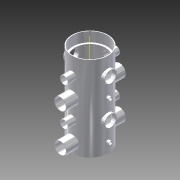
# Autodesk Inventor part: Detection Region Vacuum Collar v2
Saved by Autodesk Inventor 2015 SP1 (Build 190203100, 203)
## iProperties
Created: 2014-06-20
Part Number: Detection Region Vacuum Collar v2
Material: Aluminum 6061-AHC
Document SubType Name: Modeling
Designer: Aki
Density: 2.7 g/cm^3
Appearance: Aluminum - Dark
Author: Aki
Autodesk Inventor part; units mm, degrees
sketch "Sketch1" plane through (0, 0, 0) normal (0, 1, 0) x (-1, 0, 0)
  circle A0 centre (0, 0) radius 101.6
  circle A1 centre (0, 0) radius 97.6
  dimension "d0" = 203.2
  dimension "d3" = 195.2
  constraints: 2 centre point, 2 coincident
  measures "d0" diameter of A0
  measures "d3" diameter of A1
extrude "Extrusion2" add sketch "Sketch1" along normal blind 477.1
ref_plane "Work Plane1" through (0, 0, 101.6) normal (0, 0, 1) x (1, 0, 0)
sketch "Sketch2" plane through (0, 0, 101.6) normal (0, 0, 1) x (1, 0, 0)
  circle A0 centre (0, 57.3) radius 35.05
  circle A1 centre (0, 164.8) radius 22.25
  circle A2 centre (0, 272.3) radius 35.05
  circle A3 centre (0, 379.8) radius 22.25
  line L0 (101.6, 477.1) -> (-101.6, 477.1) projected
  line L1 (-101.6, 0) -> (101.6, 0) projected
  point P0 (0, 0)
  dimension "d7" = 70.1
  dimension "d8" = 44.5
  dimension "d9" = 70.1
  dimension "d10" = 44.5
  dimension "d11" = 97.3
  dimension "d12" = 57.3
  dimension "d13" = 215
  dimension "d14" = 215
  constraints: 4 centre point
  measures "d7" diameter of A0
  measures "d8" diameter of A1
  measures "d9" diameter of A2
  measures "d10" diameter of A3
  measures "d11" distance from line of L0 A3.centre
  measures "d12" distance from line of L1 A0.centre
  measures "d13" distance of A2.centre A0.centre
  measures "d14" distance of A3.centre A1.centre
extrude "Extrusion8" add sketch "Sketch2" against normal up to next
sketch "Sketch13" plane through (0, 0, 101.6) normal (0, 0, 1) x (1, 0, 0)
  circle A0 centre (0, 57.3) radius 35.05
  circle A1 centre (0, 164.8) radius 22.25
  circle A2 centre (0, 272.3) radius 35.05
  circle A3 centre (0, 379.8) radius 22.25
  line L0 (101.6, 477.1) -> (-101.6, 477.1) projected
  line L1 (-101.6, 0) -> (101.6, 0) projected
  point P0 (0, 0)
  dimension "d104" = 70.1
  dimension "d105" = 44.5
  dimension "d106" = 70.1
  dimension "d107" = 44.5
  dimension "d108" = 97.3
  dimension "d109" = 57.3
  dimension "d110" = 215
  dimension "d111" = 215
  constraints: 4 centre point
  measures "d104" diameter of A0
  measures "d105" diameter of A1
  measures "d106" diameter of A2
  measures "d107" diameter of A3
  measures "d108" distance from line of L0 A3.centre
  measures "d109" distance from line of L1 A0.centre
  measures "d110" distance of A2.centre A0.centre
  measures "d111" distance of A3.centre A1.centre
extrude "Extrusion9" add sketch "Sketch13" along normal blind 65
ref_plane "Work Plane2" through (0, 0, -101.6) normal (0, 0, 1) x (1, 0, 0)
sketch "Sketch3" plane through (0, 0, -101.6) normal (0, 0, 1) x (1, 0, 0)
  circle A0 centre (0, 57.3) radius 35.05
  circle A1 centre (0, 164.8) radius 22.25
  circle A2 centre (0, 272.3) radius 35.05
  circle A3 centre (0, 379.8) radius 22.25
  line L0 (101.6, 477.1) -> (-101.6, 477.1) projected
  line L1 (-101.6, 0) -> (101.6, 0) projected
  line L2 (0, 357.55) -> (0, 402.05) projected
  point P0 (0, 0)
  dimension "d18" = 70.1
  dimension "d19" = 44.5
  dimension "d20" = 70.1
  dimension "d21" = 44.5
  dimension "d22" = 97.3
  dimension "d23" = 57.3
  dimension "d24" = 215
  dimension "d25" = 215
  dimension "d26" = 0
  constraints: 4 centre point
  measures "d18" diameter of A0
  measures "d19" diameter of A1
  measures "d20" diameter of A2
  measures "d21" diameter of A3
  measures "d22" distance from line of L0 A3.centre
  measures "d23" distance from line of L1 A0.centre
  measures "d24" distance of A0.centre A2.centre
  measures "d25" distance of A3.centre A1.centre
  measures "d26" distance from line of L2 A3.centre
extrude "Extrusion10" add sketch "Sketch3" along normal up to next
sketch "Sketch14" plane through (0, 0, -101.6) normal (0, 0, 1) x (1, 0, 0)
  circle A0 centre (0, 57.3) radius 35.05
  circle A1 centre (0, 164.8) radius 22.25 projected
  circle A2 centre (0, 164.8) radius 22.25
  circle A3 centre (0, 272.3) radius 35.05
  circle A4 centre (0, 379.8) radius 22.25
  line L0 (-101.6, 0) -> (101.6, 0) projected
  line L1 (101.6, 477.1) -> (-101.6, 477.1) projected
  point P0 (0, 0)
  dimension "d116" = 70.1
  dimension "d117" = 44.5
  dimension "d118" = 70.1
  dimension "d119" = 44.5
  dimension "d120" = 57.3
  dimension "d121" = 215
  dimension "d122" = 215
  dimension "d123" = 97.3
  constraints: 4 centre point, 1 coincident
  measures "d116" diameter of A0
  measures "d117" diameter of A2
  measures "d118" diameter of A3
  measures "d119" diameter of A4
  measures "d120" distance from line of L0 A0.centre
  measures "d121" distance of A3.centre A0.centre
  measures "d122" distance of A4.centre A2.centre
  measures "d123" distance from line of L1 A4.centre
extrude "Extrusion11" add sketch "Sketch14" against normal blind 65
sketch "Sketch15" plane through (0, 379.8, -166.6) normal (0, 0, -1) x (-1, 0, 0)
  circle A0 centre (0, -322.5106) radius 34.15
  point P0 (0, -379.8)
  dimension "d126" = 68.3
  constraints: 1 centre point
  measures "d126" diameter of A0
hole "Hole8" at (0, 57.2894, -166.6) direction (0, 0, 1) diameter 61.976 end through all
sketch "Sketch16" plane through (0, 164.8, -166.6) normal (0, 0, -1) x (-1, 0, 0)
  circle A0 centre (0, 0) radius 21.35
  point P0 (0, -164.8)
  dimension "d134" = 42.7
  constraints: 1 centre point
  measures "d134" diameter of A0
hole "Hole9" at (0, 164.8, -166.6) direction (0, 0, 1) diameter 42.7 end through all
sketch "Sketch17" plane through (0, 272.3, -166.6) normal (0, 0, -1) x (-1, 0, 0)
  circle A0 centre (0, 0) radius 34.15
  point P0 (0, -272.3)
  dimension "d142" = 68.3
  constraints: 1 centre point
  measures "d142" diameter of A0
hole "Hole10" at (0, 272.3, -166.6) direction (0, 0, 1) diameter 61.976 end through all
sketch "Sketch18" plane through (0, 379.8, -166.6) normal (0, 0, -1) x (-1, 0, 0)
  circle A0 centre (0, 0) radius 21.35
  point P0 (0, -379.8)
  dimension "d150" = 42.7
  constraints: 1 centre point
  measures "d150" diameter of A0
hole "Hole11" at (0, 379.8, -166.6) direction (0, 0, 1) diameter 42.7 end through all
ref_plane "Work Plane3" through (101.6, 0, 0) normal (1, 0, 0) x (0, 1, 0)
sketch "Sketch27" plane through (101.6, 0, 0) normal (1, 0, 0) x (0, 1, 0)
  circle A0 centre (164.8, 0) radius 35.05
  circle A1 centre (379.8, 0) radius 35.05
  line L0 (477.1, -101.6) -> (477.1, 101.6) projected
  circle A2 centre (272.3, 0) radius 9.65
  circle A3 centre (57.3, 0) radius 9.65
  point P0 (0, 0)
  dimension "d204" = 70.1
  dimension "d205" = 70.1
  dimension "d206" = 97.3
  dimension "d207" = 215
  dimension "d208" = 19.3
  dimension "d209" = 19.3
  dimension "d210" = 215
  dimension "d211" = 107.5
  constraints: 4 centre point
  measures "d204" diameter of A0
  measures "d205" diameter of A1
  measures "d206" distance from line of L0 A1.centre
  measures "d207" distance of A0.centre A1.centre
  measures "d208" diameter of A2
  measures "d209" diameter of A3
  measures "d210" distance of A3.centre A2.centre
  measures "d211" distance of A2.centre A1.centre
extrude "Extrusion17" add sketch "Sketch27" against normal up to next
sketch "Sketch28" plane through (101.6, 0, 0) normal (1, 0, 0) x (0, 1, 0)
  circle A0 centre (57.3, 0) radius 9.65
  circle A1 centre (272.3, 0) radius 9.65
  circle A2 centre (164.8, 0) radius 35.05
  circle A3 centre (379.8, 0) radius 35.05
  line L0 (477.1, -101.6) -> (477.1, 101.6) projected
  point P0 (0, 0)
  dimension "d214" = 19.3
  dimension "d215" = 19.3
  dimension "d216" = 70.1
  dimension "d217" = 70.1
  dimension "d218" = 97.3
  dimension "d219" = 107.5
  dimension "d220" = 215
  dimension "d221" = 215
  constraints: 4 centre point
  measures "d214" diameter of A0
  measures "d215" diameter of A1
  measures "d216" diameter of A2
  measures "d217" diameter of A3
  measures "d218" distance from line of L0 A3.centre
  measures "d219" distance of A1.centre A3.centre
  measures "d220" distance of A2.centre A3.centre
  measures "d221" distance of A1.centre A0.centre
extrude "Extrusion18" add sketch "Sketch28" along normal blind 15
ref_plane "Work Plane8" through (-101.6, 0, 0) normal (1, 0, 0) x (0, 1, 0)
sketch "Sketch33" plane through (-101.6, 0, 0) normal (1, 0, 0) x (0, 1, 0)
  circle A0 centre (164.8, 0) radius 35.05
  circle A1 centre (379.8, 0) radius 35.05
  line L0 (477.1, -101.6) -> (477.1, 101.6) projected
  circle A2 centre (272.3, 0) radius 9.515
  circle A3 centre (57.3, 0) radius 9.65 projected
  circle A4 centre (57.3, 0) radius 9.65
  point P0 (0, 0)
  dimension "d230" = 70.1
  dimension "d231" = 70.1
  dimension "d232" = 97.3
  dimension "d233" = 215
  dimension "d234" = 19.03
  dimension "d235" = 107.5
  dimension "d236" = 19.3
  dimension "d237" = 215
  constraints: 4 centre point, 1 coincident
  measures "d230" diameter of A0
  measures "d231" diameter of A1
  measures "d232" distance from line of L0 A1.centre
  measures "d233" distance of A0.centre A1.centre
  measures "d234" diameter of A2
  measures "d235" distance of A1.centre A2.centre
  measures "d236" diameter of A4
  measures "d237" distance of A2.centre A4.centre
extrude "Extrusion19" add sketch "Sketch33" along normal up to next
sketch "Sketch34" plane through (-101.6, 0, 0) normal (1, 0, 0) x (0, 1, 0)
  circle A0 centre (379.8, 0) radius 35.05
  circle A1 centre (164.8, 0) radius 35.05
  line L0 (477.1, -101.6) -> (477.1, 101.6) projected
  arc A2 (262.785, 0) -> (281.815, 0) centre (272.3, 0) ccw projected
  circle A3 centre (272.3, 0) radius 9.65
  arc A4 (47.65, 0) -> (66.95, 0) centre (57.3, 0) ccw projected
  circle A5 centre (57.3, 0) radius 9.65
  point P0 (0, 0)
  point P1 (312.785, 0)
  point P2 (331.815, 0)
  point P3 (97.65, 0)
  point P4 (116.95, 0)
  point P5 (252.785, 0)
  point P6 (271.815, 0)
  point P7 (37.65, 0)
  point P8 (56.95, 0)
  dimension "d240" = 70.1
  dimension "d241" = 70.1
  dimension "d242" = 97.3
  dimension "d243" = 215
  dimension "d244" = 19.3
  dimension "d245" = 19.3
  dimension "d246" = 107.5
  dimension "d247" = 215
  constraints: 4 centre point, 2 coincident, 2 other
  measures "d240" diameter of A0
  measures "d241" diameter of A1
  measures "d242" distance from line of L0 A0.centre
  measures "d243" distance of A1.centre A0.centre
  measures "d244" diameter of A3
  measures "d245" diameter of A5
  measures "d246" distance of A3.centre A0.centre
  measures "d247" distance of A5.centre A3.centre
extrude "Extrusion20" add sketch "Sketch34" against normal blind 15
sketch "Sketch29" plane through (116.6, 379.8, 0) normal (1, 0, 0) x (0, 0, -1)
  circle A0 centre (0, 0) radius 34.15
  line L0 (101.6, 97.3) -> (-101.6, 97.3) projected
  point P0 (0, -379.8)
  dimension "d224" = 68.3
  dimension "d225" = 97.3
  constraints: 1 centre point
  measures "d224" diameter of A0
  measures "d225" distance from line of L0 A0.centre
sketch "Sketch30" plane through (116.6, 164.8, 0) normal (1, 0, 0) x (0, 0, -1)
  circle A0 centre (0, 0) radius 34.15
  point P0 (0, -164.8)
  dimension "d226" = 68.3
  constraints: 1 centre point
  measures "d226" diameter of A0
sketch "Sketch31" plane through (116.6, 272.3, 0) normal (1, 0, 0) x (0, 0, -1)
  circle A0 centre (0, 0) radius 8
  point P0 (0, -272.3)
  dimension "d227" = 16
  constraints: 1 centre point
  measures "d227" diameter of A0
sketch "Sketch32" plane through (116.6, 57.3, 0) normal (1, 0, 0) x (0, 0, -1)
  circle A0 centre (0, 0) radius 8
  point P0 (0, -57.3)
  dimension "d228" = 16
  constraints: 1 centre point
  measures "d228" diameter of A0
hole "Hole15" at (116.6, 379.8, 0) direction (-1, 0, 0) diameter 61.976 end through all
hole "Hole16" at (116.6, 164.8, 0) direction (-1, 0, 0) diameter 61.976 end through all
hole "Hole17" at (116.6, 272.3, 0) direction (-1, 0, 0) diameter 16 end through all
hole "Hole18" at (116.6, 57.3, 0) direction (-1, 0, 0) diameter 16 end through all
sketch "Sketch59" plane through (0, 379.8, 166.6) normal (0, 0, 1) x (1, 0, 0)
  circle A0 centre (0, 0) radius 22.25
  circle A1 centre (0, -215) radius 22.25
  line L0 (101.6, 97.3) -> (-101.6, 97.3) projected
  point P0 (0, -379.8)
  dimension "d741" = 44.5
  dimension "d742" = 44.5
  dimension "d743" = 215
  dimension "d746" = 97.3
  constraints: 2 centre point
  measures "d741" diameter of A0
  measures "d742" diameter of A1
  measures "d743" distance of A1.centre A0.centre
  measures "d746" distance from line of L0 A0.centre
extrude "Extrusion30" cut sketch "Sketch59" against normal blind 20
sketch "Sketch60" plane through (0, 379.8, -166.6) normal (0, 0, -1) x (-1, 0, 0)
  circle A0 centre (0, 0) radius 22.25
  circle A1 centre (0, -215) radius 22.25
  line L0 (101.6, 97.3) -> (-101.6, 97.3) projected
  point P0 (0, -379.8)
  dimension "d747" = 44.5
  dimension "d748" = 44.5
  dimension "d749" = 215
  dimension "d750" = 97.3
  constraints: 2 centre point
  measures "d747" diameter of A0
  measures "d748" diameter of A1
  measures "d749" distance of A0.centre A1.centre
  measures "d750" distance from line of L0 A0.centre
extrude "Extrusion31" cut sketch "Sketch60" against normal blind 20
ref_plane "Work Plane20" through (0, 16.75, 0) normal (0, 1, 0) x (-1, 0, 0)
sketch "Sketch61" plane through (0, 16.75, 0) normal (0, 1, 0) x (-1, 0, 0)
  circle A0 centre (0, 0) radius 97.6
  circle A1 centre (0, 0) radius 86.6
  dimension "d754" = 195.2
  dimension "d755" = 173.2
  constraints: 2 centre point, 2 coincident
  measures "d754" diameter of A0
  measures "d755" diameter of A1
extrude "Extrusion32" add sketch "Sketch61" along normal blind 5
ref_plane "Work Plane21" through (0, 422.1, 0) normal (0, 1, 0) x (-1, 0, 0)
sketch "Sketch62" plane through (0, 422.1, 0) normal (0, 1, 0) x (-1, 0, 0)
  circle A0 centre (0, 0) radius 97.6
  circle A1 centre (0, 0) radius 86.6
  dimension "d759" = 195.2
  dimension "d760" = 173.2
  constraints: 2 centre point, 2 coincident
  measures "d759" diameter of A0
  measures "d760" diameter of A1
extrude "Extrusion33" add sketch "Sketch62" against normal blind 5
sketch "Sketch63" plane through (0, 422.1, 0) normal (0, 1, 0) x (1, 0, 0)
  circle A0 centre (0, 90) radius 1.65
  point P0 (0, 0)
  dimension "d763" = 3.3
  dimension "d764" = 90
  constraints: 1 centre point
  measures "d763" diameter of A0
  measures "d764" distance of point (0, 0) A0.centre
sketch "Sketch64" plane through (0, 422.1, 0) normal (0, 1, 0) x (1, 0, 0)
  circle A0 centre (-63.6396, 63.6396) radius 1.65
  point P0 (0, 0)
  dimension "d765" = 3.3
  dimension "d766" = 90
  dimension "d767" = 63.6396
  constraints: 1 centre point
  measures "d765" diameter of A0
  measures "d766" distance of point (0, 0) A0.centre
  measures "d767" horizontal distance of point (0, 0) A0.centre
sketch "Sketch65" plane through (0, 422.1, 0) normal (0, 1, 0) x (1, 0, 0)
  circle A0 centre (-90, 0) radius 1.65
  point P0 (0, 0)
  dimension "d768" = 3.3
  dimension "d769" = 90
  constraints: 1 centre point
  measures "d768" diameter of A0
  measures "d769" distance of point (0, 0) A0.centre
sketch "Sketch66" plane through (0, 422.1, 0) normal (0, 1, 0) x (1, 0, 0)
  circle A0 centre (-63.6396, -63.6396) radius 1.65
  point P0 (0, 0)
  dimension "d770" = 3.3
  dimension "d771" = 90
  dimension "d772" = 63.6396
  constraints: 1 centre point
  measures "d770" diameter of A0
  measures "d771" distance of point (0, 0) A0.centre
  measures "d772" horizontal distance of point (0, 0) A0.centre
sketch "Sketch67" plane through (0, 422.1, 0) normal (0, 1, 0) x (1, 0, 0)
  circle A0 centre (0, -90) radius 1.65
  point P0 (0, 0)
  dimension "d773" = 3.3
  dimension "d774" = 90
  constraints: 1 centre point
  measures "d773" diameter of A0
  measures "d774" distance of point (0, 0) A0.centre
sketch "Sketch68" plane through (0, 422.1, 0) normal (0, 1, 0) x (1, 0, 0)
  circle A0 centre (63.6396, -63.6396) radius 1.65
  point P0 (0, 0)
  dimension "d775" = 3.3
  dimension "d776" = 90
  dimension "d777" = 63.6396
  constraints: 1 centre point
  measures "d775" diameter of A0
  measures "d776" distance of A0.centre point (0, 0)
  measures "d777" horizontal distance of A0.centre point (0, 0)
sketch "Sketch69" plane through (0, 422.1, 0) normal (0, 1, 0) x (1, 0, 0)
  circle A0 centre (90, 0) radius 1.65
  point P0 (0, 0)
  dimension "d778" = 3.3
  dimension "d779" = 90
  constraints: 1 centre point
  measures "d778" diameter of A0
  measures "d779" distance of A0.centre point (0, 0)
sketch "Sketch70" plane through (0, 422.1, 0) normal (0, 1, 0) x (1, 0, 0)
  circle A0 centre (63.6396, 63.6396) radius 1.65
  point P0 (0, 0)
  dimension "d780" = 3.3
  dimension "d781" = 90
  dimension "d782" = 63.6396
  constraints: 1 centre point
  measures "d780" diameter of A0
  measures "d781" distance of A0.centre point (0, 0)
  measures "d782" horizontal distance of A0.centre point (0, 0)
hole "Hole43" at (-63.6396, 422.1, -63.6396) direction (0, -1, 0) diameter 3.3 end through all
hole "Hole44" at (-90, 422.1, 0) direction (0, -1, 0) diameter 3.3 end through all
hole "Hole45" at (0, 422.1, -90) direction (0, -1, 0) diameter 3.3 end through all
hole "Hole46" at (-63.6396, 422.1, 63.6396) direction (0, -1, 0) diameter 3.3 end through all
hole "Hole47" at (0, 422.1, 90) direction (0, -1, 0) diameter 3.3 end through all
hole "Hole48" at (63.6396, 422.1, -63.6396) direction (0, -1, 0) diameter 3.3 end through all
hole "Hole49" at (90, 422.1, 0) direction (0, -1, 0) diameter 3.3 end through all
hole "Hole50" at (63.6396, 422.1, 63.6396) direction (0, -1, 0) diameter 3.3 end through all
body "Solid2"
